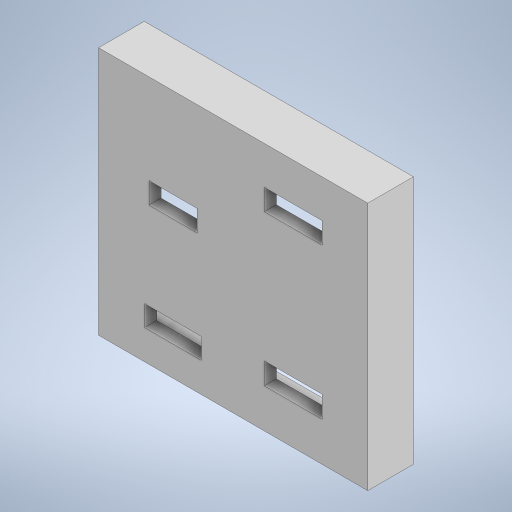
# Autodesk Inventor part: pololuAndRelayCaseTop
Saved by Autodesk Inventor 2024 (Build 280153000, 153)
## iProperties
Created: 2023-08-12
Part Number: pololuAndRelayCaseTop
Material: Generic
Document SubType Name: Modeling
Designer: 18179
Density: 1 g/cm^3
Appearance: Default
Autodesk Inventor part; units mm, degrees
ref_plane "YZ Plane" through (0, 0, 0) normal (1, 0, 0) x (0, 1, 0)
ref_plane "XZ Plane" through (0, 0, 0) normal (0, 1, 0) x (-1, 0, 0)
ref_plane "XY Plane" through (0, 0, 0) normal (0, 0, 1) x (1, 0, 0)
sketch "Sketch1" plane through (0, 0, 0) normal (0, 0, 1) x (1, 0, 0)
  point P0 (0, 0)
sketch "0" plane through (0, 0, 0) normal (0, 0, 1) x (1, 0, 0)
  line L0 (-20.32, 48.26) -> (-5.08, 48.26)
  line L1 (-5.08, 48.26) -> (-5.08, 42.672)
  line L2 (-5.08, 42.672) -> (-20.32, 42.672)
  line L3 (-20.32, 42.672) -> (-20.32, 48.26)
  line L4 (-36.95, -0.635) -> (-36.95, 4.953)
  line L5 (-36.95, 4.953) -> (-51.95, 4.953)
  line L6 (-51.95, 4.953) -> (-51.95, -0.635)
  line L7 (-51.95, -0.635) -> (-36.95, -0.635)
  line L8 (-20.32, -0.635) -> (-5.08, -0.635)
  line L9 (-5.08, -0.635) -> (-5.08, 4.953)
  line L10 (-5.08, 4.953) -> (-20.32, 4.953)
  line L11 (-20.32, 4.953) -> (-20.32, -0.635)
  line L12 (-60.96, 54.61) -> (-60.96, -3.81)
  line L13 (-60.96, -3.81) -> (3.81, -3.81)
  line L14 (3.81, -3.81) -> (3.81, 54.61)
  line L15 (3.81, 54.61) -> (-60.96, 54.61)
  line L16 (-60.96, -3.81) -> (3.81, -3.81)
  line L17 (3.81, -3.81) -> (3.81, 54.61)
  line L18 (-60.96, 54.61) -> (-60.96, -3.81)
  line L19 (-60.96, -3.81) -> (3.81, -3.81)
  line L20 (-50.8, 28.956) -> (-38.12, 28.956)
  line L21 (-38.12, 28.956) -> (-38.12, 34.544)
  line L22 (-38.12, 34.544) -> (-50.8, 34.544)
  line L23 (-50.8, 34.544) -> (-50.8, 28.956)
  line L24 (-44.45, 31.75) -> (-50.8, 31.75)
  line L25 (-50.8, 31.75) -> (-50.8, 28.956)
  line L26 (-50.8, 28.956) -> (-44.45, 28.956)
  line L27 (-44.45, 28.956) -> (-44.45, 31.75)
  line L28 (-20.32, 0.3568) -> (-36.95, 0.3568)
  line L29 (-50.8, 54.61) -> (-60.96, 54.61)
  line L30 (-5.08, -3.81) -> (3.81, -3.81)
  line L31 (3.81, -3.81) -> (3.81, 54.61)
  circle A0 centre (-54.61, 31.75) radius 1.0922
  circle A1 centre (-34.29, 31.75) radius 1.0922
  line L32 (-54.61, 31.75) -> (-34.29, 31.75)
  line L33 (3.81, 55.118) -> (-60.96, 55.118)
  line L34 (-60.96, -4.318) -> (3.81, -4.318)
  line L35 (-60.96, 55.118) -> (3.81, 55.118)
  line L36 (3.81, 55.118) -> (3.81, -4.318)
  line L37 (3.81, -4.318) -> (-60.96, -4.318)
  line L38 (-60.96, -4.318) -> (-60.96, 55.118)
  line L39 (-60.96, 58.293) -> (6.985, 58.293)
  line L40 (6.985, 58.293) -> (6.985, -4.318)
  line L41 (-64.135, 55.118) -> (-64.135, -7.493)
  line L42 (-64.135, -7.493) -> (3.81, -7.493)
  line L43 (-64.135, 55.118) -> (-60.96, 55.118)
  line L44 (-60.96, 55.118) -> (-60.96, 58.293)
  line L45 (-60.96, 58.293) -> (-64.135, 58.293)
  line L46 (-64.135, 58.293) -> (-64.135, 55.118)
  line L47 (6.985, -4.318) -> (3.81, -4.318)
  line L48 (3.81, -4.318) -> (3.81, -7.493)
  line L49 (3.81, -7.493) -> (6.985, -7.493)
  line L50 (6.985, -7.493) -> (6.985, -4.318)
  line L51 (-20.32, 2.8338) -> (-5.08, 2.8338)
  line L52 (-5.08, 2.8338) -> (-5.08, 8.5488)
  line L53 (-5.08, 8.5488) -> (-20.32, 8.5488)
  line L54 (-20.32, 8.5488) -> (-20.32, 2.8338)
  line L55 (-51.95, 0.3568) -> (-36.95, 0.3568)
  line L56 (-36.95, 0.3568) -> (-36.95, 5.832)
  line L57 (-36.95, 5.832) -> (-51.95, 5.832)
  line L58 (-51.95, 5.832) -> (-51.95, 0.3568)
  point P0 (-20.32, 51.435)
  point P1 (-5.08, 48.26)
  point P2 (-5.08, 42.672)
  point P3 (-20.32, 45.847)
  dimension "d0" = 0.508
  dimension "d1" = 0.508
  dimension "d2" = 3.175
  dimension "d3" = 3.175
  dimension "d9" = 15.24
  dimension "d10" = 5.588
  dimension "d11" = 90
  dimension "d13" = 5.588
  dimension "d14" = 5.588
  dimension "d15" = 15.24
  dimension "d16" = 15.24
  dimension "d17" = 6.35
  dimension "d18" = 5.715
  constraints: 118 end point, 12 parallel, 6 horizontal, 6 perpendicular, 4 point on line, 2 centre point, 2 other
  measures "d0" distance between parallel lines of L15 L33
  measures "d1" distance between parallel lines of L16 L34
  measures "d2" distance between parallel lines of L35 L39
  measures "d3" distance between parallel lines of L38 L41
  measures "d9" distance between parallel lines of L1 L3
  measures "d10" distance between parallel lines of L2 L0
  measures "d11" angle of L1 L2
  measures "d13" distance of L3.start L3.end
  measures "d14" distance of L1.start L1.end
  measures "d15" distance of L2.start L2.end
  measures "d16" distance of L0.start L0.end
  measures "d17" distance between parallel lines of L15 L0
  measures "d18" distance of L52.end L51.end
extrude "Extrusion1" add sketch "0" along normal blind 3.175 contours L7 L6 L55 L4 | L11 L51 L9 L8 | L15 L14 L13 L12 | L38 L33 L36 L15 | L12 L38 L34 L48 L42 L41 L43 | L13 L36 L34 L38 | L44 L39 L40 L47 L36 L14 L33 | L43 L46 L45 L44 | L47 L50 L49 L48 | A0 | A1
sketch "Sketch3" plane through (0, 0, 0) normal (0, 0, -1) x (-1, 0, 0)
  line L0 (-6.985, -7.493) -> (-6.985, 58.293) projected
  line L1 (64.135, -7.493) -> (-6.985, -7.493) projected
  line L2 (64.135, 58.293) -> (64.135, -7.493) projected
  line L3 (-6.985, 58.293) -> (64.135, 58.293) projected
  line L4 (36.95, 5.832) -> (36.95, 0.3568) projected
  line L5 (51.95, 0.3568) -> (51.95, 5.832) projected
  line L6 (50.8, 28.956) -> (50.8, 34.544) projected
  line L7 (38.12, 28.956) -> (50.8, 28.956) projected
  line L8 (38.12, 34.544) -> (38.12, 28.956) projected
  line L9 (50.8, 34.544) -> (38.12, 34.544) projected
  line L10 (20.32, 2.8338) -> (20.32, 8.5488) projected
  line L11 (5.08, 8.5488) -> (5.08, 2.8338) projected
  line L12 (-3.81, 55.118) -> (-3.81, -4.318)
  line L13 (-3.81, -4.318) -> (60.96, -4.318)
  line L14 (60.96, -4.318) -> (60.96, 55.118)
  line L15 (60.96, 55.118) -> (-3.81, 55.118)
  line L16 (5.08, 2.8338) -> (20.32, 2.8338) projected
  line L17 (20.32, 8.5488) -> (5.08, 8.5488) projected
  line L18 (36.95, 0.3568) -> (51.95, 0.3568) projected
  line L19 (51.95, 5.832) -> (36.95, 5.832) projected
  point P0 (0, 0)
  dimension "d6" = 3.175
  constraints: 8 end point, 3 other
  measures "d6" distance between parallel lines of L0 L12
extrude "Extrusion2" add sketch "Sketch3" along normal blind 8.89 contours L0 L3 L2 L1
body "Solid1"
